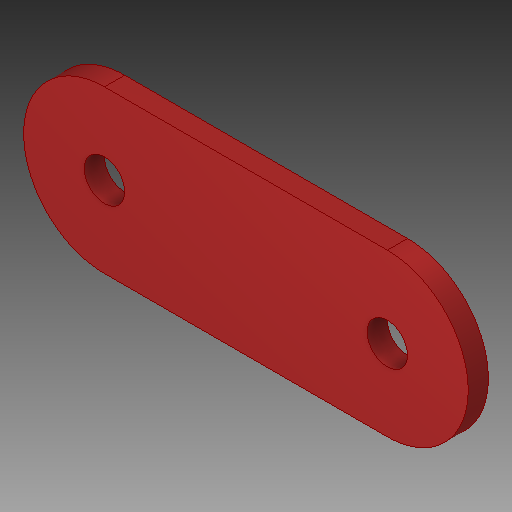
# Autodesk Inventor part: linear_slide_piece2_v2
Saved by Autodesk Inventor 2019 (Build 230136000, 136)
## iProperties
Created: 2019-01-09
Part Number: linear_slide_piece2_v2
Material: Aluminum 6061
Document SubType Name: Modeling
Designer: lebraddock
Density: 2.7 g/cm^3
Appearance: Aluminum - Flat
Mass: 13.4794 g
Surface Area: 38.0709 cm^2
Volume: 4.99237 cm^3
Author: lebraddock
Autodesk Inventor part; units mm, degrees
ref_plane "YZ Plane" through (0, 0, 0) normal (1, 0, 0) x (0, 1, 0)
ref_plane "XZ Plane" through (0, 0, 0) normal (0, 1, 0) x (-1, 0, 0)
ref_plane "XY Plane" through (0, 0, 0) normal (0, 0, 1) x (1, 0, 0)
sketch "Sketch1" plane through (0, 0, 0) normal (0, 0, 1) x (1, 0, 0)
  circle A0 centre (0, 0) radius 3.175
  arc A1 (0, -12.7) -> (0, 12.7) centre (0, 0) ccw
  line L0 (0, 12.7) -> (-9.525, 12.7)
  line L1 (0, -12.7) -> (-9.525, -12.7)
  line L2 (-9.525, 12.7) -> (-22.225, 12.7)
  line L3 (-22.225, -12.7) -> (-9.525, -12.7)
  line L4 (-22.225, 12.7) -> (0, 12.7)
  line L5 (0, -12.7) -> (-22.225, -12.7)
  circle A2 centre (-44.45, 0) radius 3.175
  arc A3 (-44.45, 12.7) -> (-44.45, -12.7) centre (-44.45, 0) ccw
  line L6 (-44.45, 12.7) -> (-34.925, 12.7)
  line L7 (-44.45, -12.7) -> (-34.925, -12.7)
  line L8 (-34.925, 12.7) -> (-22.225, 12.7)
  line L9 (-22.225, -12.7) -> (-34.925, -12.7)
  line L10 (-22.225, 12.7) -> (-44.45, 12.7)
  line L11 (-44.45, -12.7) -> (-22.225, -12.7)
  dimension "d0" = 6.35
  dimension "d5" = 25.4
  dimension "d6" = 12.7
  constraints: 24 end point, 4 centre point, 4 coincident, 4 point on circle, 2 horizontal, 2 tangent, 1 collinear, 1 parallel
  measures "d0" diameter of A0
  measures "d5" diameter of A1
  measures "d6" distance of L3.end L3.start
extrude "Extrusion1" add sketch "Sketch1" along normal blind 3.175
body "Solid1"
